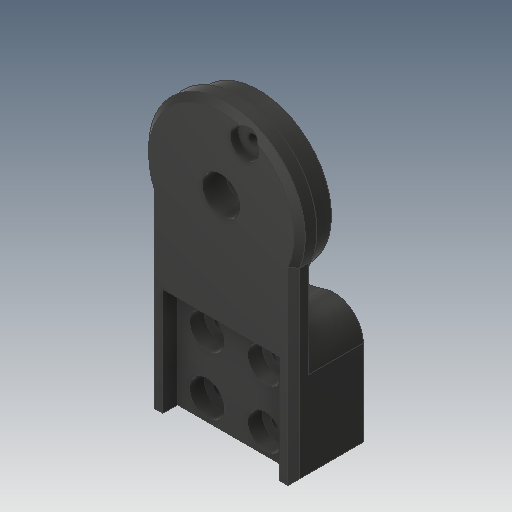
# Autodesk Inventor part: base_top
Saved by Autodesk Inventor 2020.3 (Build 243373000, 373)
## iProperties
Created: 2021-02-25
Part Number: base_top
Material: ABS Plastic
Document SubType Name: Modeling
Designer: paulg
Density: 1.06 g/cm^3
Appearance: Smooth - Black
Mass: 52.753 g
Surface Area: 185.1 cm^2
Volume: 49.767 cm^3
Author: paulg
Autodesk Inventor part; units mm, degrees
ref_plane "YZ Plane" through (0, 0, 0) normal (1, 0, 0) x (0, 1, 0)
ref_plane "XZ Plane" through (0, 0, 0) normal (0, 1, 0) x (-1, 0, 0)
ref_plane "XY Plane" through (0, 0, 0) normal (0, 0, 1) x (1, 0, 0)
sketch "Sketch1" plane through (0, 0, 0) normal (0, 0, 1) x (1, 0, 0)
  circle A0 centre (0, 0) radius 6.5
  circle A1 centre (0, 0) radius 25
  dimension "d0" = 50
  dimension "d1" = 13
  constraints: 2 centre point, 2 coincident
  measures "d0" diameter of A1
  measures "d1" diameter of A0
extrude "Extrusion1" add sketch "Sketch1" along normal blind 7
sketch "Sketch2" plane through (0, 0, 7) normal (0, 0, 1) x (1, 0, 0)
  circle A0 centre (0, 0) radius 6.5 projected
  circle A1 centre (0, 0) radius 25 projected
  circle A2 centre (0, 0) radius 27
  dimension "d4" = 2
  constraints: 1 centre point
  measures "d4" radial gap between concentric circles of A1 A2
extrude "Extrusion2" add sketch "Sketch2" along normal blind 1 contours A1 | A2
sketch "Sketch3" plane through (0, 0, 8) normal (0, 0, 1) x (1, 0, 0)
  circle A0 centre (0, 0) radius 6.5 projected
  circle A1 centre (0, 0) radius 27 projected
  line L0 (0, 0) -> (0, -42.599) construction
  circle A2 centre (0, 0) radius 27 projected
  line L1 (25, -75) -> (-25, -75)
  line L2 (-25, -75) -> (-25, -10.198)
  line L3 (-25, -10.198) -> (25, -10.198) construction
  line L4 (25, -10.198) -> (25, -75)
  line L5 (25, -75) -> (-25, -10.198) construction
  line L6 (-25, -75) -> (25, -10.198) construction
  arc A3 (-25, -10.198) -> (25, -10.198) centre (0, 0) ccw
  dimension "d7" = 50
  dimension "d8" = 75
  constraints: 14 end point, 2 midpoint, 2 parallel, 2 point on circle, 1 centre point, 1 coincident, 1 horizontal, 1 perpendicular, 1 vertical, 4 other
  measures "d7" distance of L1.start L1.end
  measures "d8" distance from line of L1 point (0, 0)
extrude "Extrusion3" add sketch "Sketch3" along normal blind 5
sketch "Sketch4" plane through (0, 0, 0) normal (0, 0, -1) x (-1, 0, 0)
  circle A0 centre (0, 0) radius 6.5 projected
  circle A1 centre (0, 0) radius 25 projected
  line L0 (15.5, -15.5) -> (-15.5, -15.5) construction
  line L1 (-15.5, -15.5) -> (-15.5, 15.5) construction
  line L2 (-15.5, 15.5) -> (15.5, 15.5) construction
  line L3 (15.5, 15.5) -> (15.5, -15.5) construction
  line L4 (15.5, -15.5) -> (-15.5, 15.5) construction
  line L5 (-15.5, -15.5) -> (15.5, 15.5) construction
  dimension "d11" = 31
  constraints: 12 end point, 4 coincident, 2 midpoint, 2 parallel, 2 perpendicular, 1 horizontal
  measures "d11" distance of L2.end L0.start
hole "Hole1" [suppressed]
fillet "Fillet1" [suppressed]
sketch "Sketch5" plane through (0, 0, 0) normal (0, 0, -1) x (-1, 0, 0)
  circle A0 centre (0, 0) radius 25 projected
  circle A1 centre (0, 0) radius 6.5 projected
  line L0 (0, 0) -> (0, 21) construction
  circle A2 centre (0, 0) radius 21 construction
  line L1 (0, 0) -> (8.0364, 19.4015) construction
  point P0 (-8.0364, 19.4015)
  point P1 (-19.4015, 8.0364)
  point P2 (-19.4015, -8.0364)
  point P3 (-8.0364, -19.4015)
  point P4 (8.0364, -19.4015)
  point P5 (19.4015, -8.0364)
  point P6 (19.4015, 8.0364)
  dimension "d20" = 22.5
  dimension "d23" = 360
  dimension "d25" = 42
  constraints: 4 end point, 2 coincident, 2 point on circle, 1 centre point, 1 vertical, 9 other
  measures "d20" angle of L1 L0
  measures "d25" diameter of A2
hole "Hole2" at (-8.0364, 19.4015, 0) at (8.0364, 19.4015, 0) at (19.4015, 8.0364, 0) at (19.4015, -8.0364, 0) at (8.0364, -19.4015, 0) at (-8.0364, -19.4015, 0) at (-19.4015, -8.0364, 0) at (-19.4015, 8.0364, 0) direction (0, 0, 1) diameter 3.3 depth 6 tip angle 118
sketch "Sketch6" plane through (0, 0, 0) normal (0, 0, -1) x (-1, 0, 0)
  circle A0 centre (0, 0) radius 7.65
  dimension "d33" = 15.3
  constraints: 1 centre point, 1 coincident
  measures "d33" diameter of A0
extrude "Extrusion4" cut sketch "Sketch6" against normal blind 5
sketch "Sketch8" plane through (0, 0, 0) normal (0, 0, -1) x (-1, 0, 0)
  circle A0 centre (0, 0) radius 10
  dimension "d40" = 20
  constraints: 1 centre point, 1 coincident
  measures "d40" diameter of A0
extrude "Extrusion6" cut sketch "Sketch8" against normal blind 1
sketch "Sketch10" plane through (0, 0, 8) normal (0, 0, -1) x (-1, 0, 0)
  arc A0 (-25, -10.198) -> (25, -10.198) centre (0, 0) ccw projected
  line L0 (-25, -10.198) -> (-25, -75) projected
  line L1 (-25, -75) -> (25, -75) projected
  line L2 (25, -75) -> (25, -10.198) projected
  circle A1 centre (0, 0) radius 6.5 projected
  arc A2 (-25, -25.9037) -> (25, -25.9037) centre (0, 0) ccw
  dimension "d46" = 36
  constraints: 2 point on circle, 2 point on line, 1 centre point, 1 coincident
  measures "d46" radius of A2
extrude "Extrusion8" add sketch "Sketch10" along normal blind 19 contours A2 L2 L1 L0
chamfer "Chamfer1" distance 2 angle 45 5 edges at (25, -42.599, 13) (-25, -42.599, 13) (0, 27, 13) (25, -75, 1) (-25, -75, 1)
sketch "Sketch12" plane through (0, 0, 13) normal (0, 0, 1) x (1, 0, 0)
  line L0 (12.0956, -60) -> (12.0956, -38) projected
  line L1 (-12.0929, -60) -> (12.0956, -60) projected
  line L2 (-12.0929, -38) -> (-12.0929, -60) projected
  line L3 (-12.0929, -38) -> (12.0956, -38) projected
  line L4 (-12.0929, -60) -> (12.0956, -60) projected
  line L5 (0.0014, -60) -> (0, 0)
  line L6 (9.0011, -43) -> (-8.9989, -43)
  line L7 (-8.9989, -43) -> (-8.9989, -55)
  line L8 (-8.9989, -55) -> (9.0011, -55)
  line L9 (9.0011, -55) -> (9.0011, -43)
  line L10 (9.0011, -43) -> (-8.9989, -55) construction
  line L11 (-8.9989, -43) -> (9.0011, -55) construction
  point P0 (0.0011, -49)
  dimension "d59" = 5
  dimension "d60" = 5
  dimension "d61" = 18
  constraints: 14 end point, 4 coincident, 3 midpoint, 2 parallel, 1 horizontal, 1 perpendicular, 1 point on line
  measures "d59" distance between parallel lines of L8 L1
  measures "d60" distance between parallel lines of L3 L6
  measures "d61" distance of L7.end L8.end
sketch "Sketch19" plane through (-23, -75, -11) normal (0, -1, 0) x (1, 0, 0)
  line L0 (2.9, 10.1) -> (43.1, 10.1)
  line L1 (43.1, 10.1) -> (43.1, -10.1)
  line L2 (43.1, -10.1) -> (2.9, -10.1)
  line L3 (2.9, -10.1) -> (2.9, 10.1)
  line L4 (46, 0) -> (0, 0) projected
  line L5 (2.9, 10.1) -> (43.1, -10.1) construction
  line L6 (43.1, 10.1) -> (2.9, -10.1) construction
  line L7 (2.9, 29.1) -> (43.1, 29.1)
  line L8 (43.1, 29.1) -> (43.1, 18.9)
  line L9 (43.1, 18.9) -> (2.9, 18.9)
  line L10 (2.9, 18.9) -> (2.9, 29.1)
  line L11 (0, 24) -> (46, 24) projected
  line L12 (2.9, 29.1) -> (43.1, 18.9) construction
  line L13 (43.1, 29.1) -> (2.9, 18.9) construction
  line L14 (3, 10.7071) -> (3.7071, 10)
  line L15 (3.7071, 10) -> (3, 9.2929)
  line L16 (3, 9.2929) -> (2.2929, 10)
  line L17 (2.2929, 10) -> (3, 10.7071)
  line L18 (2.4, 10.6) -> (3.4, 9.6) construction
  line L19 (3.4, 10.6) -> (2.4, 9.6) construction
  line L20 (43, 10.7071) -> (43.7071, 10)
  line L21 (43.7071, 10) -> (43, 9.2929)
  line L22 (43, 9.2929) -> (42.2929, 10)
  line L23 (42.2929, 10) -> (43, 10.7071)
  point P0 (23, 11)
  point P1 (23, 0)
  point P2 (23, 24)
  point P3 (42.3929, 10.1)
  point P4 (3.6071, 10.1)
  point P5 (2.9, 9.3929)
  point P6 (2.9, 0)
  point P7 (43.1, 0)
  point P8 (43.1, 9.3929)
  point P9 (43.1, 24)
  point P10 (2.9, 24)
  dimension "d104" = 40.2
  dimension "d105" = 20.2
  dimension "d106" = 40.2
  dimension "d107" = 10.2
  dimension "d108" = 1
  dimension "d109" = 1
  dimension "d110" = 1
  dimension "d111" = 1
  constraints: 44 end point, 8 midpoint, 8 parallel, 4 perpendicular, 2 horizontal
  measures "d104" distance of L1.end L2.end
  measures "d105" distance of L0.end L1.end
  measures "d106" distance of L8.end L9.end
  measures "d107" distance of L7.end L8.end
  measures "d108" distance of L15.end L16.end
  measures "d109" distance of L14.end L15.end
  measures "d110" distance of L21.end L22.end
  measures "d111" distance of L21.start L21.end
extrude "Extrusion12" cut sketch "Sketch19" against normal blind 37 contours L3 L16 L17 L14 L0 | L0 L14 L15 L16 L3 | L0 L23 L22 L21 L1 L4 L3 L16 L15 L14 | L23 L20 L21 L1 L0 | L0 L1 L21 L22 L23 | L11 L8 L9 L10
sketch "Sketch20" plane through (-20.1, -75, 7.9) normal (0, 0, 1) x (1, 0, 0)
  line L0 (0.7071, 0) -> (39.4929, 0) construction
  line L1 (20.1, 0) -> (20.1, 17) construction
  line L2 (30.1, 27) -> (10.1, 27) construction
  line L3 (10.1, 27) -> (10.1, 7) construction
  line L4 (10.1, 7) -> (30.1, 7) construction
  line L5 (30.1, 7) -> (30.1, 27) construction
  line L6 (30.1, 27) -> (10.1, 7) construction
  line L7 (10.1, 27) -> (30.1, 7) construction
  point P0 (20.1, 75)
  dimension "d114" = 17
  dimension "d115" = 20
  dimension "d116" = 20
  constraints: 14 end point, 3 midpoint, 2 parallel, 1 horizontal, 1 perpendicular, 1 vertical
  measures "d114" distance of L1.start L1.end
  measures "d115" distance of L4.end L3.end
  measures "d116" distance of L3.end L2.end
hole "Hole6" at (-10, -48, 7.9) at (10, -48, 7.9) at (10, -68, 7.9) at (-10, -68, 7.9) direction (0, 0, -1) diameter 5.5 end through all counterbore diameter 12 counterbore depth 5
fillet "Fillet3" radius 10 2 edges at (25, -25.9037, -1.5) (-25, -25.9037, -1.5)
sketch "Sketch22" plane through (0, 0, 0) normal (0, 0, -1) x (-1, 0, 0)
  circle A0 centre (-8.0364, 19.4015) radius 1.65 projected
  circle A1 centre (-8.0364, 19.4015) radius 1.7
  point P0 (0, 0)
  dimension "d131" = 3.4
  constraints: 1 centre point, 1 coincident
  measures "d131" diameter of A1
extrude "Extrusion13" cut sketch "Sketch22" against normal through all contours A0 | A1
sketch "Sketch23" plane through (0, 0, 13) normal (0, 0, 1) x (1, 0, 0)
  circle A0 centre (8.0364, 19.4015) radius 1.7 projected
  point P0 (0, 0)
  constraints: 1 coincident
hole "Hole7" at (8.0364, 19.4015, 13) direction (0, 0, -1) diameter 3.3 depth 6 tip angle 118 counterbore diameter 10 counterbore depth 3
body "Solid1"
